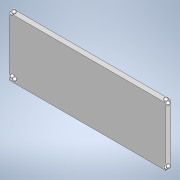
# Autodesk Inventor part: shelf120
Saved by Autodesk Inventor 2020.2 (Build 242310000, 310)
## iProperties
Created: 2020-04-20
Part Number: shelf120
Material: Generic
Document SubType Name: Modeling
Designer: Adam Nagy
Density: 1 g/cm^3
Appearance: Default
Author: Adam Nagy
Autodesk Inventor part; units mm, degrees
ref_plane "YZ Plane" through (0, 0, 0) normal (1, 0, 0) x (0, 1, 0)
ref_plane "XZ Plane" through (0, 0, 0) normal (0, 1, 0) x (-1, 0, 0)
ref_plane "XY Plane" through (0, 0, 0) normal (0, 0, 1) x (1, 0, 0)
sketch "Sketch1" plane through (0, 0, 0) normal (0, 0, 1) x (1, 0, 0)
  line L0 (0, 0) -> (1200, 0)
  line L1 (1200, 0) -> (1200, 450)
  line L2 (1200, 450) -> (0, 450)
  line L3 (0, 450) -> (0, 0)
  line L4 (3, 447) -> (1197, 447)
  line L5 (1197, 447) -> (1197, 3)
  line L6 (1197, 3) -> (3, 3)
  line L7 (3, 3) -> (3, 447)
  dimension "d8" = 1200
  dimension "d9" = 450
  dimension "d10" = 3
  constraints: 16 end point, 4 parallel, 2 perpendicular, 1 horizontal, 3 other
  measures "d8" distance between parallel lines of L1 L3
  measures "d9" distance between parallel lines of L0 L2
  measures "d10" distance between parallel lines of L2 L4
extrude "Extrusion2" add sketch "Sketch1" against normal blind 40
extrude "Extrusion3" add sketch "Sketch1" against normal blind 3 contours L3 L2 L1 L0 | L4 L5 L6 L7
sketch "Sketch2" plane through (0, 450, -40) normal (0, 1, 0) x (1, 0, 0)
  line L0 (0, -40) -> (0, 0) projected
  line L1 (1200, -40) -> (0, -40) projected
  line L2 (1200, -40) -> (1200, 0) projected
  point P0 (15, -25)
  point P1 (1185, -25)
  dimension "d22" = 15
  dimension "d23" = 15
  dimension "d24" = 15
  dimension "d25" = 15
  measures "d22" distance from line of L0 point (15, -25)
  measures "d23" distance from line of point (15, -25) L1
  measures "d24" distance from line of point (1185, -25) L1
  measures "d25" distance from line of point (1185, -25) L2
hole "Hole1" at (15, 450, -15) at (1185, 450, -15) direction (0, -1, 0) diameter 3.81 end through all
sketch "Sketch3" plane through (0, 0, -40) normal (-1, 0, 0) x (0, 0, 1)
  line L0 (40, 450) -> (40, 0) projected
  line L1 (40, 0) -> (0, 0) projected
  line L2 (40, 450) -> (0, 450) projected
  point P0 (25, 15)
  point P1 (25, 435)
  dimension "d26" = 15
  dimension "d27" = 15
  dimension "d28" = 15
  dimension "d29" = 15
  measures "d26" distance from line of L0 point (25, 15)
  measures "d27" distance from line of L1 point (25, 15)
  measures "d28" distance from line of L0 point (25, 435)
  measures "d29" distance from line of point (25, 435) L2
hole "Hole2" at (0, 15, -15) at (0, 435, -15) direction (1, 0, 0) diameter 3.81 end through all
equation "\"d8\" = Width"
equation "\"d9\" = Depth"
equation "\"d10\" = Thickness"
equation "\"d11\" = Height"
equation "\"d13\" = Thickness"
equation "\"d22\" = HoleDistance"
equation "\"d23\" = HoleDistance"
equation "\"d24\" = HoleDistance"
equation "\"d25\" = HoleDistance"
equation "\"d26\" = HoleDistance"
equation "\"d27\" = HoleDistance"
equation "\"d28\" = HoleDistance"
equation "\"d29\" = HoleDistance"
equation "\"Width\" = 1200"
equation "\"Thickness\" = 3"
equation "\"Depth\" = 450"
equation "\"Height\" = 40"
equation "\"HoleDistance\" = 15"
body "Solid2"
